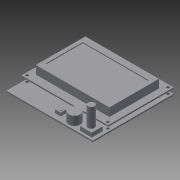
# Autodesk Inventor part: RRD Smart Graphic Controller
Saved by Autodesk Inventor 2014 SP1 (Build 180222100, 222)
## iProperties
Created: 2014-04-18
Part Number: RRD Smart Graphic Controller
Material: Generic
Document SubType Name: Modeling
Designer: Shane
Density: 1 g/cm^3
Appearance: Default
Author: Shane
Autodesk Inventor part; units mm, degrees
ref_plane "YZ Plane" through (0, 0, 0) normal (1, 0, 0) x (0, 1, 0)
ref_plane "XZ Plane" through (0, 0, 0) normal (0, 1, 0) x (-1, 0, 0)
sketch "Sketch1" plane through (0, 0, 0) normal (0, 0, 1) x (1, 0, 0)
  line L0 (0, 0) -> (93.5, 0)
  line L1 (93.5, 0) -> (93.5, 87.5)
  line L2 (93.5, 87.5) -> (0, 87.5)
  line L3 (0, 87.5) -> (0, 0)
  line L4 (3, 84.5) -> (90.5, 84.5) construction
  line L5 (90.5, 84.5) -> (90.5, 19.5) construction
  line L6 (90.5, 19.5) -> (3, 19.5) construction
  line L7 (3, 19.5) -> (3, 84.5) construction
  circle A0 centre (3, 84.5) radius 1.5
  circle A1 centre (90.5, 84.5) radius 1.5
  circle A2 centre (90.5, 19.5) radius 1.5
  circle A3 centre (3, 19.5) radius 1.5
  dimension "d0" = 93.5
  dimension "d1" = 87.5
  dimension "d2" = 87.5
  dimension "d3" = 65
  dimension "d4" = 3
  dimension "d5" = 3
  dimension "d6" = 3
  constraints: 16 end point, 4 centre point, 4 coincident, 4 parallel, 3 equal radius, 2 horizontal, 2 perpendicular
  measures "d0" distance of L2.end L1.end
  measures "d1" distance of L1.end L0.end
  measures "d2" distance of L5.end L6.end
  measures "d3" distance of L4.end L5.end
  measures "d4" distance between parallel lines of L4 L2
  measures "d5" distance between parallel lines of L7 L3
  measures "d6" diameter of A0
extrude "Extrusion1" add sketch "Sketch1" against normal blind 1.5
sketch "Sketch2" plane through (0, 0, -1.5) normal (0, 0, -1) x (-1, 0, 0)
  line L0 (0, 0) -> (0, 87.5) projected
  line L1 (0, 87.5) -> (-93.5, 87.5) projected
  line L2 (0, 65.5) -> (-26, 65.5)
  line L3 (-26, 65.5) -> (-26, 38.5)
  line L4 (-26, 38.5) -> (0, 38.5)
  line L5 (0, 38.5) -> (0, 65.5)
  dimension "d9" = 22
  dimension "d10" = 26
  dimension "d11" = 27
  constraints: 8 end point, 2 parallel, 1 horizontal, 1 perpendicular, 1 point on line
  measures "d9" distance between parallel lines of L2 L1
  measures "d10" distance of L2.start L2.end
  measures "d11" distance of L2.end L3.end
extrude "Extrusion2" add sketch "Sketch2" along normal blind 3.5
sketch "Sketch3" plane through (0, 0, -1.5) normal (0, 0, -1) x (-1, 0, 0)
  line L0 (0, 65.5) -> (0, 87.5) projected
  line L1 (0, 87.5) -> (-93.5, 87.5) projected
  line L2 (-42, 81.5) -> (-21.5, 81.5)
  line L3 (-21.5, 81.5) -> (-21.5, 72)
  line L4 (-21.5, 72) -> (-42, 72)
  line L5 (-42, 72) -> (-42, 81.5)
  line L6 (-72.5, 81.5) -> (-52, 81.5)
  line L7 (-52, 81.5) -> (-52, 72)
  line L8 (-52, 72) -> (-72.5, 72)
  line L9 (-72.5, 72) -> (-72.5, 81.5)
  dimension "d14" = 21.5
  dimension "d15" = 6
  dimension "d16" = 9.5
  dimension "d17" = 20.5
  dimension "d18" = 10
  dimension "d19" = 6
  constraints: 16 end point, 4 parallel, 2 equal length, 2 horizontal, 2 perpendicular
  measures "d14" distance between parallel lines of L0 L3
  measures "d15" distance between parallel lines of L2 L1
  measures "d16" distance of L2.end L3.end
  measures "d17" distance of L2.start L2.end
  measures "d18" distance between parallel lines of L7 L5
  measures "d19" distance between parallel lines of L1 L6
extrude "Extrusion3" add sketch "Sketch3" along normal blind 19
ref_plane "Work Plane1" through (0, 0, 4.6) normal (0, 0, 1) x (1, 0, 0)
sketch "Sketch4" plane through (0, 0, 4.6) normal (0, 0, 1) x (1, 0, 0)
  line L0 (0, 0) -> (0, 16.5) construction
  line L1 (0, 16.5) -> (93.5, 16.5)
  line L2 (93.5, 16.5) -> (93.5, 87.5)
  line L3 (93.5, 87.5) -> (0, 87.5)
  line L4 (0, 87.5) -> (0, 16.5)
  line L5 (3, 84.5) -> (90.5, 84.5) construction
  line L6 (90.5, 84.5) -> (90.5, 19.5) construction
  line L7 (90.5, 19.5) -> (3, 19.5) construction
  line L8 (3, 19.5) -> (3, 84.5) construction
  circle A0 centre (3, 84.5) radius 1.5
  circle A1 centre (90.5, 84.5) radius 1.5
  circle A2 centre (90.5, 19.5) radius 1.5
  circle A3 centre (3, 19.5) radius 1.5
  dimension "d23" = 16.5
  dimension "d24" = 93.5
  dimension "d25" = 71
  dimension "d26" = 87.5
  dimension "d27" = 65
  dimension "d28" = 3
  dimension "d29" = 3
  dimension "d30" = 3
  constraints: 18 end point, 4 centre point, 4 coincident, 4 parallel, 3 equal radius, 2 horizontal, 2 perpendicular, 1 vertical
  measures "d23" distance of L0.start L0.end
  measures "d24" distance of L3.end L2.end
  measures "d25" distance of L2.end L1.end
  measures "d26" distance of L6.end L7.end
  measures "d27" distance of L5.end L6.end
  measures "d28" distance between parallel lines of L3 L5
  measures "d29" distance between parallel lines of L4 L8
  measures "d30" diameter of A0
extrude "Extrusion4" add sketch "Sketch4" along normal blind 1.5
sketch "Sketch5" plane through (0, 0, 6.1) normal (0, 0, 1) x (1, 0, 0)
  line L0 (0, 16.5) -> (93.5, 16.5) projected
  line L1 (93.5, 16.5) -> (93.5, 87.5) projected
  line L2 (93.5, 87.5) -> (0, 87.5) projected
  line L3 (0, 87.5) -> (0, 16.5) projected
  line L4 (7, 78.5) -> (86.5, 78.5)
  line L5 (86.5, 78.5) -> (86.5, 25)
  line L6 (86.5, 25) -> (7, 25)
  line L7 (7, 25) -> (7, 78.5)
  point P0 (0, 0)
  dimension "d33" = 9
  dimension "d34" = 7
  dimension "d35" = 7
  dimension "d36" = 8.5
  dimension "d37" = 53.5
  constraints: 8 end point, 2 parallel, 1 horizontal, 1 perpendicular
  measures "d33" distance between parallel lines of L2 L4
  measures "d34" distance between parallel lines of L1 L5
  measures "d35" distance between parallel lines of L3 L7
  measures "d36" distance between parallel lines of L0 L6
  measures "d37" distance of L4.end L5.end
extrude "Extrusion5" add sketch "Sketch5" along normal blind 9 contours L4 L5 L6 L7
sketch "Sketch6" plane through (7, 25, 6.1) normal (-1, 0, 0) x (0, 0, 1)
  line L0 (0, 0) -> (0, 53.5) projected
  line L1 (0, 53.5) -> (9, 53.5) projected
  line L2 (0, 49) -> (3.5, 49)
  line L3 (3.5, 49) -> (3.5, 5.9)
  line L4 (3.5, 5.9) -> (0, 5.9)
  line L5 (0, 5.9) -> (0, 49)
  point P0 (-6.1, -25)
  dimension "d40" = 3.5
  dimension "d41" = 43.1
  dimension "d42" = 4.5
  constraints: 8 end point, 2 parallel, 1 horizontal, 1 perpendicular, 1 point on line
  measures "d40" distance of L3.end L4.end
  measures "d41" distance of L2.end L3.end
  measures "d42" distance between parallel lines of L1 L2
extrude "Extrusion6" add sketch "Sketch6" along normal blind 5
sketch "Sketch7" plane through (0, 0, 0) normal (0, 0, 1) x (1, 0, 0)
  line L0 (47.5, 11.3) -> (53.5, 11.3)
  line L1 (53.5, 11.3) -> (53.5, 5.3)
  line L2 (53.5, 5.3) -> (47.5, 5.3)
  line L3 (47.5, 5.3) -> (47.5, 11.3)
  line L4 (0, 0) -> (93.5, 0) projected
  line L5 (93.5, 0) -> (93.5, 87.5) projected
  dimension "d45" = 6
  dimension "d46" = 6
  dimension "d52" = 40
  dimension "d53" = 5.3
  constraints: 8 end point, 2 parallel, 1 horizontal, 1 perpendicular
  measures "d45" distance of L1.end L2.end
  measures "d46" distance of L0.end L1.end
  measures "d52" distance between parallel lines of L5 L1
  measures "d53" distance between parallel lines of L4 L2
extrude "Extrusion7" add sketch "Sketch7" along normal blind 3.5
sketch "Sketch8" plane through (0, 0, 3.5) normal (0, 0, 1) x (1, 0, 0)
  circle A0 centre (50.4777, 8.3572) radius 1.75
  point P0 (0, 0)
  dimension "d49" = 3.5
  constraints: 1 centre point
  measures "d49" diameter of A0
extrude "Extrusion8" add sketch "Sketch8" along normal blind 0.5
sketch "Sketch9" plane through (0, 0, 0) normal (0, 0, 1) x (1, 0, 0)
  line L0 (0, 0) -> (93.5, 0) projected
  line L1 (93.5, 0) -> (93.5, 87.5) projected
  circle A0 centre (65.5, 8.3) radius 6.25
  dimension "d54" = 12.5
  dimension "d55" = 28
  dimension "d56" = 8.3
  constraints: 1 centre point
  measures "d54" diameter of A0
  measures "d55" distance from line of L1 A0.centre
  measures "d56" distance from line of L0 A0.centre
extrude "Extrusion9" add sketch "Sketch9" along normal blind 9.5
sketch "Sketch10" plane through (0, 0, 0) normal (0, 0, 1) x (1, 0, 0)
  line L0 (0, 0) -> (93.5, 0) projected
  line L1 (93.5, 0) -> (93.5, 87.5) projected
  line L2 (77.3, 14.3) -> (90, 14.3)
  line L3 (90, 14.3) -> (90, 2.3)
  line L4 (90, 2.3) -> (77.3, 2.3)
  line L5 (77.3, 2.3) -> (77.3, 14.3)
  line L6 (77.3, 14.3) -> (90, 2.3) construction
  line L7 (90, 14.3) -> (77.3, 2.3) construction
  point P0 (83.65, 8.3)
  dimension "d59" = 12.7
  dimension "d60" = 12
  dimension "d61" = 3.5
  dimension "d62" = 2.3
  constraints: 12 end point, 2 midpoint, 2 parallel, 1 horizontal, 1 perpendicular
  measures "d59" distance of L3.end L4.end
  measures "d60" distance of L2.end L3.end
  measures "d61" distance between parallel lines of L1 L3
  measures "d62" distance between parallel lines of L0 L4
extrude "Extrusion10" add sketch "Sketch10" along normal blind 4.5
sketch "Sketch11" plane through (0, 0, 4.5) normal (0, 0, 1) x (1, 0, 0)
  circle A0 centre (83.65, 8.3) radius 3.5
  point P0 (0, 0)
  dimension "d65" = 7
  constraints: 1 centre point
  measures "d65" diameter of A0
extrude "Extrusion11" add sketch "Sketch11" along normal blind 20.3
sketch "Sketch12" plane through (0, 0, 15.1) normal (0, 0, 1) x (1, 0, 0)
  line L0 (86.5, 78.5) -> (7, 78.5) projected
  line L1 (7, 78.5) -> (7, 25) projected
  line L2 (7, 25) -> (86.5, 25) projected
  line L3 (86.5, 25) -> (86.5, 78.5) projected
  line L4 (11, 71.75) -> (82.5, 71.75)
  line L5 (82.5, 71.75) -> (82.5, 31.75)
  line L6 (82.5, 31.75) -> (11, 31.75)
  line L7 (11, 31.75) -> (11, 71.75)
  point P0 (0, 0)
  dimension "d68" = 71.5
  dimension "d69" = 40
  dimension "d70" = 6.75
  dimension "d71" = 6.75
  dimension "d72" = 4
  dimension "d73" = 4
  constraints: 8 end point, 2 parallel, 1 horizontal, 1 perpendicular
  measures "d68" distance of L5.end L6.end
  measures "d69" distance of L4.end L5.end
  measures "d70" distance between parallel lines of L0 L4
  measures "d71" distance between parallel lines of L2 L6
  measures "d72" distance between parallel lines of L1 L7
  measures "d73" distance between parallel lines of L3 L5
extrude "Extrusion12" cut sketch "Sketch12" against normal blind 1 contours L4 L5 L6 L7
body "Solid1"
